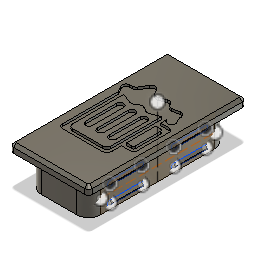
frame plug (Autodesk Fusion 360 design; units mm, degrees)
Autodesk Fusion 360 part; units mm, degrees
sketch "Sketch1" plane through (0, 0, 0) normal (0, 1, 0) x (1, 0, 0)
  line L0 (0, 0) -> (20, 0)
  line L1 (20, 0) -> (20, -40)
  line L2 (20, -40) -> (0, -40)
  line L3 (0, -40) -> (0, 0)
  line L4 (2.6828, -15.061) -> (2.6828, -29.3493)
  line L5 (3.6828, -30.3493) -> (13.6966, -30.3493)
  line L6 (14.9966, -29.0493) -> (14.9966, -15.1348)
  line L7 (14.9966, -16.6829) -> (17.0881, -16.6829)
  line L8 (18.0881, -17.6829) -> (18.0881, -25.6449)
  line L9 (17.0881, -26.6449) -> (14.9966, -26.6449)
  line L10 (5.0451, -17.9656) -> (5.0451, -25.8205)
  arc A0 (5.0451, -25.8205) -> (6.8451, -25.8205) centre (5.9451, -25.8205) ccw
  line L11 (6.8451, -25.8205) -> (6.8451, -17.9656)
  arc A1 (6.8451, -17.9656) -> (5.0451, -17.9656) centre (5.9451, -17.9656) ccw
  line L12 (5.9451, -17.9656) -> (5.9451, -25.8205) construction
  line L13 (8.0451, -17.9656) -> (8.0451, -25.8205)
  arc A2 (8.0451, -25.8205) -> (9.8451, -25.8205) centre (8.9451, -25.8205) ccw
  line L14 (9.8451, -25.8205) -> (9.8451, -17.9656)
  arc A3 (9.8451, -17.9656) -> (8.0451, -17.9656) centre (8.9451, -17.9656) ccw
  line L15 (11.0451, -17.9656) -> (11.0451, -25.8205)
  arc A4 (11.0451, -25.8205) -> (12.8451, -25.8205) centre (11.9451, -25.8205) ccw
  line L16 (12.8451, -25.8205) -> (12.8451, -17.9656)
  arc A5 (12.8451, -17.9656) -> (11.0451, -17.9656) centre (11.9451, -17.9656) ccw
  line L17 (2.6828, -15.061) -> (3.9828, -15.061)
  line L18 (3.9828, -15.061) -> (3.9828, -28.0493)
  line L19 (4.9828, -29.0493) -> (12.6966, -29.0493)
  line L20 (13.6966, -28.0493) -> (13.6966, -15.1348)
  line L21 (14.9966, -17.9829) -> (16.3481, -17.9829)
  line L22 (16.7881, -18.4229) -> (16.7881, -24.9049)
  line L23 (16.3481, -25.3449) -> (14.9966, -25.3449)
  arc A6 (2.6828, -29.3493) -> (3.6828, -30.3493) centre (3.6828, -29.3493) ccw
  arc A7 (13.6966, -30.3493) -> (14.9966, -29.0493) centre (13.6966, -29.0493) ccw
  arc A8 (17.0881, -26.6449) -> (18.0881, -25.6449) centre (17.0881, -25.6449) ccw
  arc A9 (18.0881, -17.6829) -> (17.0881, -16.6829) centre (17.0881, -17.6829) ccw
  arc A10 (3.9828, -28.0493) -> (4.9828, -29.0493) centre (4.9828, -28.0493) ccw
  arc A11 (12.6966, -29.0493) -> (13.6966, -28.0493) centre (12.6966, -28.0493) ccw
  arc A12 (16.7881, -18.4229) -> (16.3481, -17.9829) centre (16.3481, -18.4229) ccw
  arc A13 (16.3481, -25.3449) -> (16.7881, -24.9049) centre (16.3481, -24.9049) ccw
  line L24 (2.6828, -15.061) -> (1.8313, -13.7109)
  line L25 (2.6771, -12.1774) -> (3.2757, -12.1774)
  line L26 (4.1256, -11.7043) -> (5.3287, -9.7639)
  line L27 (7.0244, -9.7574) -> (7.8154, -11.0115)
  line L28 (9.0257, -11.4092) -> (10.705, -10.7519)
  line L29 (12.0007, -11.3186) -> (12.0667, -11.4873)
  line L30 (13.1934, -12.1036) -> (15.0176, -11.74)
  line L31 (16.213, -12.7207) -> (16.213, -12.9404)
  line L32 (16.328, -13.406) -> (16.91, -14.5123)
  line L33 (13.6966, -15.1348) -> (11.3896, -16.0377)
  line L34 (10.5387, -15.9802) -> (9.3409, -15.3135)
  line L35 (8.2825, -15.3671) -> (7.4688, -15.9347)
  line L36 (6.5364, -16.0473) -> (3.9828, -15.061)
  arc A14 (7.0244, -9.7574) -> (5.3287, -9.7639) centre (6.1786, -10.2909) ccw
  arc A15 (3.2757, -12.1774) -> (4.1256, -11.7043) centre (3.2757, -11.1774) ccw
  arc A16 (7.8154, -11.0115) -> (9.0257, -11.4092) centre (8.6612, -10.478) ccw
  arc A17 (12.0007, -11.3186) -> (10.705, -10.7519) centre (11.0695, -11.6831) ccw
  arc A18 (12.0667, -11.4873) -> (13.1934, -12.1036) centre (12.998, -11.1228) ccw
  arc A19 (16.213, -12.7207) -> (15.0176, -11.74) centre (15.213, -12.7207) ccw
  arc A20 (16.213, -12.9404) -> (16.328, -13.406) centre (17.213, -12.9404) ccw
  arc A21 (15.1164, -15.3955) -> (16.91, -14.5123) centre (16.025, -14.9779) ccw
  arc A22 (10.5387, -15.9802) -> (11.3896, -16.0377) centre (11.0251, -15.1065) ccw
  arc A23 (9.3409, -15.3135) -> (8.2825, -15.3671) centre (8.8546, -16.1873) ccw
  arc A24 (6.5364, -16.0473) -> (7.4688, -15.9347) centre (6.8967, -15.1145) ccw
  arc A25 (2.6771, -12.1774) -> (1.8313, -13.7109) centre (2.6771, -13.1774) ccw
  line L37 (13.6966, -15.1348) -> (14.9966, -15.1348)
  line L38 (15.1164, -15.3955) -> (14.9966, -15.1348)
  dimension "d1" = 20
  dimension "d2" = 40
  dimension "d3" = 1.8
  dimension "d6" = 6
  dimension "d7" = 0
  dimension "d10" = 1
  dimension "d11" = 1.3
  dimension "d12" = 1
  dimension "d13" = 0.44
  dimension "d14" = 1
  dimension "d15" = 10.0137
  dimension "d16" = 1.3
  dimension "d17" = 1.3
  dimension "d18" = 1.3
  dimension "d47" = 1.3
  dimension "d48" = 1.3
  dimension "d49" = 1.3
  constraint horizontal L0
  constraint vertical L1
  constraint horizontal L2
  constraint vertical L3
  constraint coincident L0.start L3.end
  constraint parallel L3 L4
  constraint perpendicular L3 L5
  constraint perpendicular L5 L6
  constraint coincident L6 L7.start
  constraint perpendicular L6 L7
  constraint perpendicular L7 L8
  constraint coincident L6 L9.end
  constraint perpendicular L6 L9
  constraint tangent L10 A0
  constraint tangent A0 L11
  constraint parallel L10 L11
  constraint tangent L11 A1
  constraint tangent L10 A1
  constraint vertical L12
  constraint perpendicular L4 L17
  constraint tangent L4 A6
  constraint tangent L5 A6
  constraint tangent L6 A7
  constraint tangent L5 A7
  constraint tangent L8 A8
  constraint tangent L9 A8
  constraint tangent L7 A9
  constraint tangent L8 A9
  constraint equal A8 A9
  constraint parallel L4 L18
  constraint parallel L5 L19
  constraint parallel L6 L20
  constraint tangent L18 A10
  constraint tangent L19 A10
  constraint equal A8 A10
  constraint tangent L19 A11
  constraint tangent L20 A11
  constraint equal A8 A11
  constraint parallel L7 L21
  constraint parallel L8 L22
  constraint parallel L9 L23
  constraint tangent L21 A12
  constraint tangent L22 A12
  constraint tangent L22 A13
  constraint tangent L23 A13
  constraint equal A12 A13
  constraint perpendicular L4 L25
  constraint parallel L24 L27
  constraint perpendicular L28 L29
  constraint perpendicular L17 L31
  constraint parallel L28 L33
  constraint tangent L26 A14
  constraint tangent L27 A14
  constraint tangent L25 A15
  constraint tangent L26 A15
  constraint equal A14 A15
  constraint tangent L27 A16
  constraint tangent L28 A16
  constraint equal A14 A16
  constraint tangent L28 A17
  constraint tangent L29 A17
  constraint equal A14 A17
  constraint tangent L29 A18
  constraint tangent L30 A18
  constraint equal A14 A18
  constraint tangent L30 A19
  constraint tangent L31 A19
  constraint equal A14 A19
  constraint tangent L31 A20
  constraint tangent L32 A20
  constraint equal A14 A20
  constraint tangent L32 A21
  constraint equal A14 A21
  constraint tangent L33 A22
  constraint tangent L34 A22
  constraint equal A14 A22
  constraint tangent L34 A23
  constraint tangent L35 A23
  constraint equal A14 A23
  constraint tangent L35 A24
  constraint tangent L36 A24
  constraint equal A14 A24
  constraint tangent L24 A25
  constraint tangent L25 A25
  constraint equal A14 A25
  constraint perpendicular L6 L37
  constraint tangent A21 L38
  constraint coincident L17.end L18.start
  constraint coincident L6 L21.start
  constraint coincident L6 L23.end
  measures "d1" distance of L0.start L0.end
  measures "d2" distance of L0.start L2.end
  measures "d3" diameter of A0
  measures "d10" radius of A6
  measures "d11" radius of A7
  measures "d12" radius of A8
  measures "d13" radius of A12
  measures "d14" radius of A14
  measures "d15" distance of L5.start L5.end
  measures "d16" distance of L4.start L17.end
  measures "d17" distance of L6.end L20.end
  measures "d18" vertical distance of L5.start L19.start
  measures "d47" distance of L7.start L21.start
  measures "d48" horizontal distance of L8.end L22.end
  measures "d49" distance of L9.end L23.end
extrude "Extrude1" add sketch "Sketch1" against normal blind 2 contours L0 L1 L2 L3 | L4 L5 L6 L17 L18 L19 L20 A6 A7 A10 A11 L37 | L17 L24 L25 L26 L27 L28 L29 L30 L31 L32 L33 L34 L35 L36 A14 A15 A16 A17 A18 A19 A20 A21 A22 A23 A24 A25 L37 L38 | L18 L19 L20 A10 A11 L33 L34 L35 L36 A22 A23 A24 | L6 L7 L8 L9 L21 L22 L23 A8 A9 A12 A13 | L6 L21 L22 L23 A12 A13 | L10 A0 L11 A1 | L13 A2 L14 A3 | L15 A4 L16 A5
extrude "Extrude2" cut sketch "Sketch1" against normal blind 0.6 contours L4 L5 L6 L17 L18 L19 L20 A6 A7 A10 A11 L37 | L17 L24 L25 L26 L27 L28 L29 L30 L31 L32 L33 L34 L35 L36 A14 A15 A16 A17 A18 A19 A20 A21 A22 A23 A24 A25 L37 L38 | L6 L7 L8 L9 L21 L22 L23 A8 A9 A12 A13 | L10 A0 L11 A1 | L13 A2 L14 A3 | L15 A4 L16 A5
fillet "Fillet1" radius 1 4 edges at (0, -1, 40) (20, -1, 40) (0, -1, 0) (20, -1, 0)
chamfer "Chamfer1" distance 0.7 angle 45 8 edges at (0, 0, 20) (0.2929, 0, 0.2929) (10, 0, 0) (19.7071, 0, 0.2929) (20, 0, 20) (19.7071, 0, 39.7071) (10, 0, 40) (0.2929, 0, 39.7071)
sketch "Sketch2" plane through (0, -2, 0) normal (0, -1, 0) x (1, 0, 0)
  arc A0 (19, 0) -> (20, 1) centre (19, 1) ccw
  line L0 (20, 1) -> (20, 39)
  arc A1 (20, 39) -> (19, 40) centre (19, 39) ccw
  line L1 (19, 40) -> (1, 40)
  arc A2 (1, 40) -> (0, 39) centre (1, 39) ccw
  line L2 (0, 39) -> (0, 1)
  arc A3 (0, 1) -> (1, 0) centre (1, 1) ccw
  line L3 (1, 0) -> (19, 0)
  line L4 (5.5, 37.5) -> (14.5, 37.5)
  line L5 (17.5, 34.5) -> (17.5, 5.5)
  line L6 (14.5, 2.5) -> (5.5, 2.5)
  line L7 (2.5, 5.5) -> (2.5, 34.5)
  arc A4 (5.5, 37.5) -> (2.5, 34.5) centre (5.5, 34.5) ccw
  arc A5 (17.5, 34.5) -> (14.5, 37.5) centre (14.5, 34.5) ccw
  arc A6 (2.5, 5.5) -> (5.5, 2.5) centre (5.5, 5.5) ccw
  arc A7 (14.5, 2.5) -> (17.5, 5.5) centre (14.5, 5.5) ccw
  line L8 (4.1, 5.5) -> (4.1, 34.5)
  arc A8 (5.5, 35.9) -> (4.1, 34.5) centre (5.5, 34.5) ccw
  line L9 (5.5, 35.9) -> (14.5, 35.9)
  arc A9 (15.9, 34.5) -> (14.5, 35.9) centre (14.5, 34.5) ccw
  line L10 (15.9, 34.5) -> (15.9, 5.5)
  arc A10 (14.5, 4.1) -> (15.9, 5.5) centre (14.5, 5.5) ccw
  line L11 (14.5, 4.1) -> (5.5, 4.1)
  arc A11 (4.1, 5.5) -> (5.5, 4.1) centre (5.5, 5.5) ccw
  point P0 (2.5, 37.5)
  point P1 (17.5, 2.5)
  point P2 (0, 40)
  point P3 (20, 0)
  dimension "d26" = 2.5
  dimension "d27" = 2.5
  dimension "d28" = 2.5
  dimension "d29" = 2.5
  dimension "d30" = 3
  dimension "d31" = 3
  dimension "d32" = 3
  dimension "d33" = 3
  dimension "d34" = 1.6
  constraint horizontal L4
  constraint vertical L5
  constraint horizontal L6
  constraint vertical L7
  constraint coincident P0 L4
  constraint coincident P0 L7
  constraint tangent L4 A4
  constraint tangent L7 A4
  constraint tangent L4 A5
  constraint tangent L5 A5
  constraint tangent L6 A6
  constraint tangent L7 A6
  constraint coincident P1 L5
  constraint coincident P1 L6
  constraint tangent L5 A7
  constraint tangent L6 A7
  measures "d26" vertical distance of P0 P2
  measures "d27" horizontal distance of P0 P2
  measures "d28" horizontal distance of P1 P3
  measures "d29" vertical distance of P1 P3
  measures "d30" radius of A4
  measures "d31" radius of A5
  measures "d32" radius of A6
  measures "d33" radius of A7
extrude "Extrude3" add sketch "Sketch2" along normal blind 8 contours L4 L5 L6 L7 A4 A5 A6 A7
sketch "Sketch3" plane through (17.5, 0, 0) normal (1, 0, 0) x (0, 0, -1)
  line L0 (-5.5, -2) -> (-34.5, -2)
  line L1 (-34.5, -2) -> (-34.5, -10)
  line L2 (-34.5, -10) -> (-5.5, -10)
  line L3 (-5.5, -10) -> (-5.5, -2)
  line L4 (-32.118, -4.8483) -> (-24.0663, -4.8483)
  arc A0 (-24.0663, -4.8483) -> (-24.0663, -3.6483) centre (-24.0663, -4.2483) ccw
  line L5 (-24.0663, -3.6483) -> (-32.118, -3.6483)
  arc A1 (-32.118, -3.6483) -> (-32.118, -4.8483) centre (-32.118, -4.2483) ccw
  line L6 (-32.118, -4.2483) -> (-24.0663, -4.2483) construction
  line L7 (-20, -10) -> (-20, 7.5595) construction
  line L8 (-34.5, -6.3904) -> (-5.5, -6.3904) construction
  line L9 (-24.0663, -9.1325) -> (-32.118, -9.1325)
  arc A2 (-32.118, -7.9325) -> (-32.118, -9.1325) centre (-32.118, -8.5325) ccw
  line L10 (-32.118, -7.9325) -> (-24.0663, -7.9325)
  arc A3 (-24.0663, -9.1325) -> (-24.0663, -7.9325) centre (-24.0663, -8.5325) ccw
  arc A4 (-15.9337, -7.9325) -> (-15.9337, -9.1325) centre (-15.9337, -8.5325) ccw
  line L11 (-15.9337, -9.1325) -> (-7.882, -9.1325)
  arc A5 (-7.882, -9.1325) -> (-7.882, -7.9325) centre (-7.882, -8.5325) ccw
  line L12 (-7.882, -7.9325) -> (-15.9337, -7.9325)
  line L13 (-7.882, -4.2483) -> (-15.9337, -4.2483) construction
  line L14 (-7.882, -4.8483) -> (-15.9337, -4.8483)
  arc A6 (-15.9337, -3.6483) -> (-15.9337, -4.8483) centre (-15.9337, -4.2483) ccw
  arc A7 (-7.882, -4.8483) -> (-7.882, -3.6483) centre (-7.882, -4.2483) ccw
  line L15 (-15.9337, -3.6483) -> (-7.882, -3.6483)
  dimension "d37" = 1.2
  constraint tangent L4 A0
  constraint tangent A0 L5
  constraint parallel L4 L5
  constraint tangent L5 A1
  constraint tangent L4 A1
  constraint horizontal L6
  constraint midpoint L2 L7.start
  constraint perpendicular L2 L7
  constraint symmetric L4.start L8 A2.start
  constraint symmetric L4.end L8 L10.end
  constraint symmetric A0.end L8 L9.start
  constraint symmetric L5.end L8 L9.end
  constraint symmetric A0 L8 A3
  constraint symmetric A1 L8 A2
  constraint symmetric L4.start L7 L14.start
  constraint symmetric L4.end L7 L14.end
  constraint symmetric A0.end L7 A6.start
  constraint symmetric L5.end L7 A7.end
  constraint symmetric A0 L7 A6
  constraint symmetric A1 L7 A7
  constraint symmetric L7 L9.start A4.end
  constraint symmetric L7 L9.end L11.end
  constraint symmetric L7 A2.start A5.end
  constraint symmetric L7 A2 A5
  constraint symmetric L7 L10.end A4.start
  constraint symmetric L7 A3 A4
  measures "d37" diameter of A0
extrude "Extrude4" add sketch "Sketch3" along normal blind 0.5 contours L4 A0 L5 A1 | L9 A2 L10 A3 | A4 L11 A5 L12 | L14 A6 A7 L15
chamfer "Chamfer2" distance 0.5 angle 45 16 edges at (18, -3.6483, 28.0922) (18, -4.2483, 32.718) (18, -4.8483, 28.0922) (18, -4.2483, 23.4663) (18, -7.9325, 28.0922) (18, -8.5325, 32.718) (18, -9.1325, 28.0922) (18, -8.5325, 23.4663) (18, -7.9325, 11.9078) (18, -8.5325, 16.5337) (18, -9.1325, 11.9078) (18, -8.5325, 7.282) (18, -3.6483, 11.9078) (18, -4.2483, 16.5337) (18, -4.8483, 11.9078) (18, -4.2483, 7.282)
ref_plane "WorkPlane1" through (10, -6, 20) normal (1, 0, 0) x (0, 0, 1)
mirror "Mirror2" about plane through (10, -6, 20) normal (1, 0, 0) of "Extrude4", "Chamfer2"
